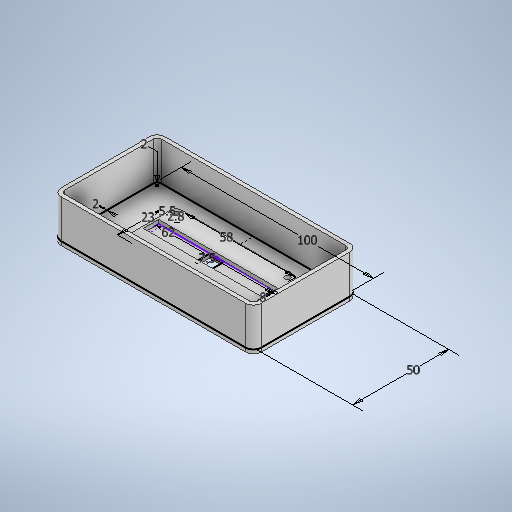
# Autodesk Inventor part: RemoteCasing
Saved by Autodesk Inventor 2025 (Build 290162000, 162)
## iProperties
Created: 2025-02-27
Part Number: RemoteCasing
Material: Generic
Document SubType Name: Modeling
Designer: tvoko
Density: 1 g/cm^3
Appearance: Default
Author: tvoko
Autodesk Inventor part; units mm, degrees
ref_plane "YZ Plane" through (0, 0, 0) normal (1, 0, 0) x (0, 1, 0)
ref_plane "XZ Plane" through (0, 0, 0) normal (0, 1, 0) x (-1, 0, 0)
ref_plane "XY Plane" through (0, 0, 0) normal (0, 0, 1) x (1, 0, 0)
sketch "Sketch1" plane through (0, 0, 0) normal (0, 1, 0) x (-1, 0, 0)
  line L0 (-2, 0) -> (-98, 0)
  line L1 (-100, -2) -> (-100, -48)
  line L2 (-98, -50) -> (-2, -50)
  line L3 (0, -48) -> (0, -2)
  arc A0 (-2, -50) -> (0, -48) centre (-2, -48) ccw
  arc A1 (-100, -48) -> (-98, -50) centre (-98, -48) ccw
  arc A2 (-98, 0) -> (-100, -2) centre (-98, -2) ccw
  arc A3 (0, -2) -> (-2, 0) centre (-2, -2) ccw
  line L4 (2, -2) -> (2, -48)
  arc A4 (-2, -52) -> (2, -48) centre (-2, -48) ccw
  line L5 (-2, -52) -> (-98, -52)
  arc A5 (-102, -48) -> (-98, -52) centre (-98, -48) ccw
  line L6 (-102, -48) -> (-102, -2)
  arc A6 (-98, 2) -> (-102, -2) centre (-98, -2) ccw
  line L7 (-98, 2) -> (-2, 2)
  arc A7 (2, -2) -> (-2, 2) centre (-2, -2) ccw
  line L8 (-21.2889, -15.4236) -> (-79.2889, -15.4236) construction
  line L9 (-79.2889, -15.4236) -> (-79.2889, -38.4236) construction
  line L10 (-79.2889, -38.4236) -> (-21.2889, -38.4236) construction
  line L11 (-21.2889, -38.4236) -> (-21.2889, -15.4236) construction
  circle A8 centre (-21.2889, -38.4236) radius 1.4
  circle A9 centre (-79.2889, -38.4236) radius 1.4
  circle A10 centre (-79.2889, -15.4236) radius 1.4
  circle A11 centre (-21.2889, -15.4236) radius 1.4
  circle A12 centre (-21.2889, -38.4236) radius 2.75
  circle A13 centre (-79.2889, -38.4236) radius 2.75
  circle A14 centre (-79.2889, -15.4236) radius 2.75
  circle A15 centre (-21.2889, -15.4236) radius 2.75
  line L12 (-18.5389, -38.4236) -> (-18.5389, -15.4236)
  line L13 (-21.2889, -12.6736) -> (-79.2889, -12.6736)
  line L14 (-82.0389, -15.4236) -> (-82.0389, -38.4236)
  line L15 (-79.2889, -41.1736) -> (-21.2889, -41.1736)
  line L16 (-19.61, -31.0936) -> (-81.61, -31.0936)
  line L17 (-81.61, -31.0936) -> (-81.61, -23.0936)
  line L18 (-81.61, -23.0936) -> (-19.61, -23.0936)
  line L19 (-19.61, -23.0936) -> (-19.61, -31.0936)
  line L20 (-21.2889, -35.6736) -> (-79.2889, -35.6736) construction
  line L21 (-21.2889, -18.1736) -> (-79.2889, -18.1736) construction
  line L22 (-46.25, -30.8183) -> (-53.75, -30.8183)
  line L23 (-53.75, -30.8183) -> (-53.75, -23.3183)
  line L24 (-53.75, -23.3183) -> (-46.25, -23.3183)
  line L25 (-46.25, -23.3183) -> (-46.25, -30.8183)
  line L26 (-50, -50) -> (-50, 0) construction
  point P0 (0, 0)
  point P1 (-100, -50)
  point P2 (-100, 0)
  point P3 (0, -50)
  point P4 (-50, -30.8183)
  dimension "d0" = 50
  dimension "d1" = 100
  dimension "d2" = 2
  dimension "d3" = 2
  dimension "d4" = 2.8
  dimension "d5" = 58
  dimension "d6" = 23
  dimension "d7" = 5.5
  dimension "d8" = 62
  dimension "d9" = 8
  dimension "d10" = 7.5
  constraints: 54 end point, 28 point on circle, 16 centre point, 16 tangent, 13 point on line, 10 parallel, 9 equal radius, 8 coincident, 7 perpendicular, 4 horizontal, 3 midpoint, 7 other
  measures "d0" distance of point (-100, 0) point (-100, -50)
  measures "d1" distance of point (-100, -50) point (0, -50)
  measures "d2" radius of A0
  measures "d3" distance between parallel lines of L3 L4
  measures "d4" diameter of A8
  measures "d5" distance of L9.end L10.end
  measures "d6" distance of L10.end L8.start
  measures "d7" diameter of A12
  measures "d8" distance of L16.start L16.end
  measures "d9" distance of L16.end L17.end
  measures "d10" distance of L24.end L22.start
extrude "Extrusion1" add sketch "Sketch1" against normal blind 2 contours A3 L3 A0 L2 A1 L1 A2 L0 | L4 A4 L5 A5 L6 A6 L7 A7 | A8 | A9 | A10 | A11 | A12 | A12 L15 A13 L14 A14 L13 A15 L12 | A15 | A13 | A14 | L16 L17 L18 L19
extrude "Extrusion2" add sketch "Sketch1" along normal blind 20 contours L4 A4 L5 A5 L6 A6 L7 A7
extrude "Extrusion3" add sketch "Sketch1" along normal blind 2 contours A12 | A12 L15 A13 L14 A14 L13 A15 L12 | A15 | A13 | A14
body "Solid1"
